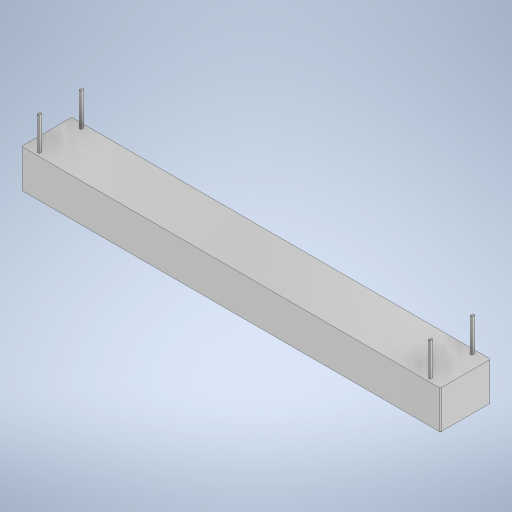
# Autodesk Inventor part: Body
Saved by Autodesk Inventor 2023 (Build 270158000, 158)
## iProperties
Created: 2024-03-19
Part Number: Body
Material: Generic
Document SubType Name: Modeling
Designer: noname
Density: 1 g/cm^3
Appearance: Aluminum - Polished
Author: noname
Autodesk Inventor part; units mm, degrees
ref_plane "YZ Plane" through (0, 0, 0) normal (1, 0, 0) x (0, 1, 0)
ref_plane "XZ Plane" through (0, 0, 0) normal (0, 1, 0) x (-1, 0, 0)
ref_plane "XY Plane" through (0, 0, 0) normal (0, 0, 1) x (1, 0, 0)
sketch "Sketch3" plane through (0, 0, 0) normal (0, 1, 0) x (-1, 0, 0)
  line L0 (37.5, 4.5) -> (-37.5, 4.5)
  line L1 (-37.5, 4.5) -> (-37.5, -4.5)
  line L2 (-37.5, -4.5) -> (37.5, -4.5)
  line L3 (37.5, -4.5) -> (37.5, 4.5)
  line L4 (37.5, 4.5) -> (-37.5, -4.5) construction
  line L5 (-37.5, 4.5) -> (37.5, -4.5) construction
  point P0 (0, 0)
  dimension "d0" = 75
  dimension "d1" = 9
  constraints: 12 end point, 2 midpoint, 2 parallel, 1 horizontal, 1 perpendicular
  measures "d0" distance between parallel lines of L1 L3
  measures "d1" distance between parallel lines of L0 L2
extrude "Extrusion1" add sketch "Sketch3" along normal blind 7
sketch "Sketch4" plane through (0, 7, 0) normal (0, 1, 0) x (1, 0, 0)
  line L0 (-37.5, 4.5) -> (-37.5, -4.5) projected
  line L1 (-37.5, 0) -> (37.5, 0)
  line L2 (37.5, -4.5) -> (37.5, 4.5) projected
  line L3 (37.5, 4.5) -> (-37.5, 4.5) projected
  line L4 (0, 4.5) -> (0, -4.5)
  line L5 (-37.5, -4.5) -> (37.5, -4.5) projected
  line L6 (-35.2, 3.45) -> (-34.8, 3.45)
  line L7 (-34.8, 3.45) -> (-34.8, 4.05)
  line L8 (-34.8, 4.05) -> (-35.2, 4.05)
  line L9 (-35.2, 4.05) -> (-35.2, 3.45)
  line L10 (-35.2, 3.45) -> (-34.8, 4.05) construction
  line L11 (-34.8, 3.45) -> (-35.2, 4.05) construction
  line L12 (-35.2, -3.45) -> (-34.8, -3.45)
  line L13 (-34.8, -3.45) -> (-34.8, -4.05)
  line L14 (-34.8, -4.05) -> (-35.2, -4.05)
  line L15 (-35.2, -4.05) -> (-35.2, -3.45)
  line L16 (-35.2, -3.45) -> (-34.8, -4.05) construction
  line L17 (-34.8, -3.45) -> (-35.2, -4.05) construction
  line L18 (35.2, 3.45) -> (34.8, 3.45)
  line L19 (34.8, 3.45) -> (34.8, 4.05)
  line L20 (34.8, 4.05) -> (35.2, 4.05)
  line L21 (35.2, 4.05) -> (35.2, 3.45)
  line L22 (35.2, 3.45) -> (34.8, 4.05) construction
  line L23 (34.8, 3.45) -> (35.2, 4.05) construction
  line L24 (35.2, -3.45) -> (34.8, -3.45)
  line L25 (34.8, -3.45) -> (34.8, -4.05)
  line L26 (34.8, -4.05) -> (35.2, -4.05)
  line L27 (35.2, -4.05) -> (35.2, -3.45)
  line L28 (35.2, -3.45) -> (34.8, -4.05) construction
  line L29 (34.8, -3.45) -> (35.2, -4.05) construction
  point P0 (0, 0)
  point P1 (-35, 3.75)
  point P2 (-35, -3.75)
  point P3 (35, 3.75)
  point P4 (35, -3.75)
  dimension "d7" = 0.6
  dimension "d8" = 0.4
  dimension "d9" = 7.5
  dimension "d10" = 70
  constraints: 52 end point, 15 symmetric about line, 6 midpoint, 2 parallel, 1 horizontal, 1 perpendicular
  measures "d7" distance between parallel lines of L6 L8
  measures "d8" distance between parallel lines of L7 L9
  measures "d9" diameter of point (-35, 3.75) L1
  measures "d10" diameter of point (-35, 3.75) L4
extrude "Extrusion2" add sketch "Sketch4" along normal blind 6 contours L9 L8 L7 L6 | L12 L13 L14 L15 | L18 L19 L20 L21 | L27 L26 L25 L24
sketch "Sketch5" plane through (0, 0, 0) normal (0, -1, 0) x (1, 0, 0)
  line L0 (-33.3, -1) -> (33.3, -1)
  line L1 (33.3, -1) -> (33.3, 1)
  line L2 (33.3, 1) -> (-33.3, 1)
  line L3 (-33.3, 1) -> (-33.3, -1)
  line L4 (-33.3, -1) -> (33.3, 1) construction
  line L5 (33.3, -1) -> (-33.3, 1) construction
  point P0 (0, 0)
  dimension "d13" = 66.6
  dimension "d14" = 2
  constraints: 12 end point, 2 midpoint, 2 parallel, 1 horizontal, 1 perpendicular
  measures "d13" distance between parallel lines of L1 L3
  measures "d14" distance between parallel lines of L0 L2
extrude "Extrusion3" cut sketch "Sketch5" against normal blind 5
sketch "Sketch6" plane through (0, 0, 0) normal (0, -1, 0) x (1, 0, 0)
  circle A0 centre (-35.5, 0) radius 1
  line L0 (37.5, -4.5) -> (-37.5, -4.5) projected
  line L1 (0, -4.5) -> (0, 4.5)
  line L2 (-37.5, 4.5) -> (37.5, 4.5) projected
  circle A1 centre (35.5, 0) radius 1
  point P0 (0, 0)
  point P1 (0, 0)
  dimension "d17" = 2
  dimension "d18" = 71
  constraints: 3 midpoint, 2 centre point, 2 end point, 1 horizontal alignment, 1 symmetric about line, 1 other
  measures "d17" diameter of A0
  measures "d18" distance of A1.centre A0.centre
extrude "Extrusion4" cut sketch "Sketch6" against normal blind 5
thread "Thread1" size "M2x0.4" class "6H" standard "ANSI Metric M Profile" length 5
thread "Thread2" size "M2x0.4" class "6H" standard "ANSI Metric M Profile" length 5
chamfer "Chamfer1" distance 0.2 angle 45 8 edges at (-37.5, 3.5, -4.5) (-37.5, 3.5, 4.5) (37.5, 3.5, -4.5) (37.5, 3.5, 4.5) (0, 0, -4.5) (37.5, 0, 0) (0, 0, 4.5) (-37.5, 0, 0)
chamfer "Chamfer2" distance 0.1 angle 45 32 edges at (-34.8, 10, -3.45) (-35.2, 10, -3.45) (-34.8, 10, -4.05) (-35.2, 10, -4.05) (-35.2, 13, -3.75) (-34.8, 13, -3.75) (-35, 13, -4.05) (-35, 13, -3.45) (-34.8, 10, 4.05) (-34.8, 13, 3.75) (-35, 13, 4.05) (-35.2, 13, 3.75) (-35.2, 10, 4.05) (-34.8, 10, 3.45) (-35, 13, 3.45) (-35.2, 10, 3.45) (34.8, 13, 3.75) (35, 13, 4.05) (35.2, 13, 3.75) (34.8, 10, 4.05) (35.2, 10, 4.05) (35, 13, 3.45) (34.8, 10, 3.45) (35.2, 10, 3.45) (34.8, 10, -3.45) (35, 13, -3.45) (35.2, 10, -3.45) (34.8, 13, -3.75) (34.8, 10, -4.05) (35.2, 13, -3.75) (35.2, 10, -4.05) (35, 13, -4.05)
body "Solid1"
